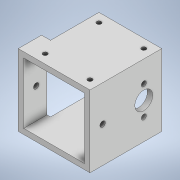
# Autodesk Inventor part: ギヤボックス２右
Saved by Autodesk Inventor 2021.3 (Build 253353000, 353)
## iProperties
Created: 2021-11-06
Part Number: ギヤボックス２右
Material: 一般
Document SubType Name: Modeling
Designer: gilte
Density: 1 g/cm^3
Appearance: 既定
Author: gilte
Autodesk Inventor part; units mm, degrees
ref_plane "YZ Plane" through (0, 0, 0) normal (1, 0, 0) x (0, 1, 0)
ref_plane "XZ Plane" through (0, 0, 0) normal (0, 1, 0) x (-1, 0, 0)
ref_plane "XY Plane" through (0, 0, 0) normal (0, 0, 1) x (1, 0, 0)
sketch "スケッチ1" plane through (0, 0, 0) normal (0, 0, 1) x (1, 0, 0)
  line L0 (0, 0) -> (40, 0)
  line L1 (40, 0) -> (40, 40)
  line L2 (40, 40) -> (0, 40)
  line L3 (0, 40) -> (0, 0)
  dimension "d0" = 40
  dimension "d1" = 40
  constraints: 8 end point, 2 parallel, 1 horizontal, 1 perpendicular
  measures "d0" distance of L2.end L1.end
  measures "d1" distance of L1.end L0.end
extrude "押し出し1" add sketch "スケッチ1" along normal blind 40
shell "シェル1" thickness 3 removed faces 2 at (26.6667, 13.3333, 0) at (26.6667, 13.3333, 40)
sketch "スケッチ2" plane through (0, 0, 0) normal (-1, 0, 0) x (0, 0, 1)
  line L0 (0, 40) -> (0, 0) projected
  line L1 (0, 40) -> (40, 40) projected
  line L2 (0, 0) -> (27, 0)
  line L3 (27, 0) -> (27, 40)
  line L4 (27, 40) -> (0, 40)
  line L5 (0, 40) -> (0, 0)
  dimension "d5" = 27
  constraints: 8 end point, 2 parallel, 1 horizontal, 1 perpendicular, 1 point on line
  measures "d5" distance of L4.end L3.end
extrude "押し出し2" cut sketch "スケッチ2" against normal blind 5
sketch "スケッチ3" plane through (0, 0, 40) normal (-1, 0, 0) x (0, 0, 1)
  circle A0 centre (-7, 20) radius 1.5
  line L0 (0, 40) -> (0, 0) projected
  line L1 (-13, 0) -> (0, 0) projected
  point P0 (-40, 0)
  dimension "d8" = 3
  dimension "d9" = 7
  dimension "d10" = 20
  constraints: 1 centre point
  measures "d8" diameter of A0
  measures "d9" distance from line of L0 A0.centre
  measures "d10" distance from line of L1 A0.centre
hole "穴1" at (0, 20, 33) direction (1, 0, 0) diameter 3 end through all
sketch "スケッチ4" plane through (0, 40, 40) normal (0, 1, 0) x (1, 0, 0)
  line L0 (35, 35) -> (10, 35)
  line L1 (10, 35) -> (10, 5)
  line L2 (10, 5) -> (35, 5)
  line L3 (35, 5) -> (35, 35)
  line L4 (40, 40) -> (5, 40) projected
  line L5 (40, 40) -> (40, 0) projected
  point P0 (0, 40)
  dimension "d18" = 25
  dimension "d19" = 30
  dimension "d20" = 5
  dimension "d21" = 5
  constraints: 8 end point, 2 parallel, 1 horizontal, 1 perpendicular
  measures "d18" distance of L2.end L1.end
  measures "d19" distance of L1.end L0.end
  measures "d20" distance between parallel lines of L4 L0
  measures "d21" distance between parallel lines of L5 L3
hole "穴2" at (10, 40, 5) at (35, 40, 5) at (35, 40, 35) at (10, 40, 35) direction (0, -1, 0) diameter 2.459 depth 3 thread size "M3x0.5" class "6H" standard "ISO Metric profile"
sketch "スケッチ5" plane through (40, 0, 0) normal (1, 0, 0) x (0, 0, -1)
  line L0 (0, 0) -> (-40, 0) projected
  line L1 (0, 0) -> (0, 40) projected
  point P0 (-10, 12)
  point P1 (-10, 28)
  dimension "d29" = 16
  dimension "d32" = 12
  dimension "d33" = 10
  dimension "d34" = 10
  measures "d29" distance of point (-10, 12) point (-10, 28)
  measures "d32" distance from line of L0 point (-10, 12)
  measures "d33" distance from line of L1 point (-10, 12)
  measures "d34" distance from line of L1 point (-10, 28)
hole "穴3" at (40, 28, 10) at (40, 12, 10) direction (-1, 0, 0) diameter 2.8 depth 3
sketch "スケッチ6" plane through (40, 0, 0) normal (1, 0, 0) x (0, 0, -1)
  circle A0 centre (-10, 20) radius 5
  line L0 (0, 0) -> (0, 40) projected
  line L1 (0, 0) -> (-40, 0) projected
  dimension "d42" = 10
  dimension "d43" = 10
  dimension "d44" = 20
  constraints: 1 centre point
  measures "d42" diameter of A0
  measures "d43" distance from line of L0 A0.centre
  measures "d44" distance from line of L1 A0.centre
extrude "押し出し3" cut sketch "スケッチ6" against normal blind 5
